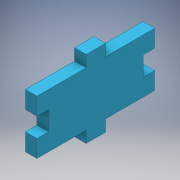
# Autodesk Inventor part: back
Saved by Autodesk Inventor 2018 (Build 220112000, 112)
## iProperties
Created: 2020-03-13
Part Number: back
Material: Genérico
Document SubType Name: Modeling
Designer: joser
Density: 1 g/cm^3
Appearance: Turquesa
Author: joser
Autodesk Inventor part; units mm, degrees
ref_plane "YZ Plane" through (0, 0, 0) normal (1, 0, 0) x (0, 1, 0)
ref_plane "XZ Plane" through (0, 0, 0) normal (0, 1, 0) x (-1, 0, 0)
ref_plane "XY Plane" through (0, 0, 0) normal (0, 0, 1) x (1, 0, 0)
sketch "Boceto2" plane through (0, 0, 0) normal (1, 0, 0) x (0, 1, 0)
  line L0 (12.7595, 3) -> (17.7595, 3)
  line L1 (0, -4.5) -> (3, -4.5)
  line L2 (3, -4.5) -> (3, -9.5)
  line L3 (3, -9.5) -> (0, -9.5)
  line L4 (0, -14) -> (0, -9.5)
  line L5 (0, -4.5) -> (0, 0)
  line L6 (0, 0) -> (12.7595, 0)
  line L7 (12.7595, 0) -> (12.7595, 3)
  line L8 (17.7595, 0) -> (30.519, 0)
  line L9 (17.7595, 0) -> (17.7595, 3)
  line L10 (17.7595, -14) -> (17.7595, -17)
  line L11 (17.7595, -17) -> (12.7595, -17)
  line L12 (12.7595, -17) -> (12.7595, -14)
  line L13 (30.519, -14) -> (17.7595, -14)
  line L14 (12.7595, -14) -> (0, -14)
  line L15 (30.519, -4.5) -> (27.519, -4.5)
  line L16 (27.519, -4.5) -> (27.519, -9.5)
  line L17 (27.519, -9.5) -> (30.519, -9.5)
  line L18 (30.519, 0) -> (30.519, -4.5)
  line L19 (30.519, -9.5) -> (30.519, -14)
  dimension "d0" = 30.519
  dimension "d2" = 5
  dimension "d3" = 3
  dimension "d4" = 3
  dimension "d5" = 5
  dimension "d6" = 20
  dimension "d7" = 3
  constraints: 40 end point, 17 perpendicular, 10 equal length, 6 parallel, 2 horizontal, 1 coincident, 1 collinear, 1 vertical
  measures "d0" distance of L13.start L4.start
  measures "d2" distance between parallel lines of L3 L1
  measures "d3" distance between parallel lines of L4 L2
  measures "d4" distance of L0.end L8.start
  measures "d5" distance of L0.start L0.end
  measures "d6" distance between parallel lines of L0 L11
  measures "d7" distance of L15.start L15.end
extrude "Extrusión1" add sketch "Boceto2" along normal blind 3
